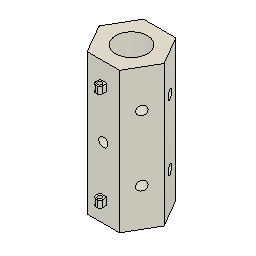
Pen_Holder (Autodesk Fusion 360 design; units mm, degrees)
Autodesk Fusion 360 part; units mm, degrees
sketch "Sketch1" plane through (0, 0, 0) normal (0, 1, 0) x (1, 0, 0)
  line L0 (2.3672, -5.715) -> (5.715, -2.3672)
  line L1 (5.715, -2.3672) -> (5.715, 2.3672)
  line L2 (5.715, 2.3672) -> (2.3672, 5.715)
  line L3 (2.3672, 5.715) -> (-2.3672, 5.715)
  line L4 (-2.3672, 5.715) -> (-5.715, 2.3672)
  line L5 (-5.715, 2.3672) -> (-5.715, -2.3672)
  line L6 (-5.715, -2.3672) -> (-2.3672, -5.715)
  line L7 (-2.3672, -5.715) -> (2.3672, -5.715)
  circle A0 centre (0, 0) radius 5.715
  line L8 (5.8659, -10.16) -> (11.7318, 0)
  line L9 (11.7318, 0) -> (5.8659, 10.16)
  line L10 (5.8659, 10.16) -> (-5.8659, 10.16)
  line L11 (-5.8659, 10.16) -> (-11.7318, 0)
  line L12 (-11.7318, 0) -> (-5.8659, -10.16)
  line L13 (-5.8659, -10.16) -> (5.8659, -10.16)
  dimension "d1" = 5.715
  dimension "d2" = 10.16
  constraint coincident A0.centre origin
  constraint tangent L7 A0
  measures "d1" distance of A0.centre L7
  measures "d2" distance of A0.centre L13
extrude "Extrude1" add sketch "Sketch1" along normal blind 50.8 contours L0 L7 A0 | L0 L1 A0 | L6 L7 A0 | L1 L2 A0 | L5 L6 A0 | L2 L3 A0 | L4 L5 A0 | L3 L4 A0 | L8 L9 L10 L11 L12 L13
sketch "Sketch2" plane through (-8.7988, 0, 5.08) normal (-0.866025, 0, 0.5) x (0.5, 0, 0.866025)
  line L0 (-5.8659, 0) -> (5.8659, 0)
  line L1 (5.8659, 0) -> (5.8659, 50.8)
  line L2 (5.8659, 50.8) -> (-5.8659, 50.8)
  line L3 (-5.8659, 50.8) -> (-5.8659, 0)
  line L4 (0, 0) -> (0, 50.8) construction
  circle A0 centre (0, 13.6652) radius 1.651
  circle A1 centre (0, 37.1348) radius 1.651
  dimension "d5" = 3.302
  dimension "d6" = 3.302
  dimension "d7" = 13.6652
  dimension "d8" = 13.6652
  constraint coincident L4.start origin
  constraint midpoint L2 L4.end
  constraint coincident L4 A0.centre
  constraint coincident L4 A1.centre
  measures "d5" diameter of A0
  measures "d6" diameter of A1
  measures "d7" distance of L2 A1.centre
  measures "d8" distance of L0 A0.centre
extrude "Extrude2" cut sketch "Sketch2" against normal blind 8.0264 contours A0 | A1
sketch "Sketch3" plane through (0, 0, 10.16) normal (0, 0, 1) x (1, 0, 0)
  line L0 (-5.8659, 0) -> (5.8659, 0)
  line L1 (5.8659, 0) -> (5.8659, 50.8)
  line L2 (5.8659, 50.8) -> (-5.8659, 50.8)
  line L3 (-5.8659, 50.8) -> (-5.8659, 0)
  line L4 (-1.27, 6.35) -> (1.27, 6.35)
  line L5 (1.27, 6.35) -> (1.27, 8.89)
  line L6 (1.27, 8.89) -> (-1.27, 8.89)
  line L7 (-1.27, 8.89) -> (-1.27, 6.35)
  line L8 (0, 50.8) -> (0, 0) construction
  line L9 (0, 8.89) -> (0, 6.35) construction
  line L10 (-5.8659, 25.4) -> (5.8659, 25.4) construction
  line L11 (1.27, 44.45) -> (1.27, 41.91)
  line L12 (1.27, 41.91) -> (-1.27, 41.91)
  line L13 (-1.27, 44.45) -> (1.27, 44.45)
  line L14 (-1.27, 41.91) -> (-1.27, 44.45)
  dimension "d11" = 2.54
  dimension "d12" = 2.54
  dimension "d13" = 6.35
  constraint horizontal L4
  constraint vertical L5
  constraint horizontal L6
  constraint vertical L7
  constraint midpoint L2 L8.start
  constraint coincident L8.end origin
  constraint midpoint L6 L9.start
  constraint midpoint L4 L9.end
  constraint collinear L8 L9
  constraint midpoint L3 L10.start
  constraint midpoint L1 L10.end
  constraint symmetric L4.start L10 L13.start
  constraint symmetric L4.end L10 L11.start
  constraint symmetric L5.end L10 L11.end
  constraint symmetric L6.end L10 L12.end
  measures "d11" distance of L4.start L4.end
  measures "d12" distance of L4.start L6.end
  measures "d13" distance of L0 L4
extrude "Extrude3" add sketch "Sketch3" along normal blind 2.54 contours L4 L5 L6 L7 | L11 L12 L13 L14
sketch "Sketch4" plane through (0, 6.35, 0) normal (0, -1, 0) x (1, 0, 0)
  line L0 (-1.27, 10.16) -> (1.27, 10.16)
  line L1 (1.27, 10.16) -> (1.27, 12.7)
  line L2 (1.27, 12.7) -> (-1.27, 12.7)
  line L3 (-1.27, 12.7) -> (-1.27, 10.16)
  line L4 (0, 12.7) -> (0, 10.16) construction
  line L5 (-1.27, 11.43) -> (1.27, 11.43)
  circle A0 centre (0, 11.43) radius 0.762
  dimension "d16" = 1.524
  constraint midpoint L2 L4.start
  constraint midpoint L0 L4.end
  constraint midpoint L3 L5.start
  constraint midpoint L1 L5.end
  constraint midpoint L5 A0.centre
  measures "d16" diameter of A0
extrude "Extrude5" cut sketch "Sketch4" against normal blind 65.6107 contours L5 A0 | L5 A0
fillet "Fillet1" radius 0.8382 4 edges at (-1.27, 7.62, 12.7) (1.27, 7.62, 12.7) (-1.27, 43.18, 12.7) (1.27, 43.18, 12.7)
sketch "Sketch5" plane through (-8.7988, 0, -5.08) normal (-0.866025, 0, -0.5) x (-0.5, 0, 0.866025)
  line L0 (-5.8659, 0) -> (5.8659, 0)
  line L1 (5.8659, 0) -> (5.8659, 50.8)
  line L2 (5.8659, 50.8) -> (-5.8659, 50.8)
  line L3 (-5.8659, 50.8) -> (-5.8659, 0)
  line L4 (0, 50.8) -> (0, 0) construction
  line L5 (5.8659, 25.4) -> (-5.8659, 25.4) construction
  line L6 (1.27, 44.45) -> (-1.27, 44.45)
  line L7 (-1.27, 44.45) -> (-1.27, 41.91)
  line L8 (-1.27, 41.91) -> (1.27, 41.91)
  line L9 (1.27, 41.91) -> (1.27, 44.45)
  line L10 (0, 41.91) -> (0, 44.45) construction
  line L11 (-1.27, 8.89) -> (1.27, 8.89)
  line L12 (1.27, 8.89) -> (1.27, 6.35)
  line L13 (1.27, 6.35) -> (-1.27, 6.35)
  line L14 (-1.27, 6.35) -> (-1.27, 8.89)
  dimension "d22" = 2.54
  dimension "d23" = 2.54
  dimension "d24" = 6.35
  constraint midpoint L2 L4.start
  constraint coincident L4.end origin
  constraint midpoint L1 L5.start
  constraint midpoint L3 L5.end
  constraint horizontal L6
  constraint vertical L7
  constraint horizontal L8
  constraint vertical L9
  constraint midpoint L8 L10.start
  constraint midpoint L6 L10.end
  constraint collinear L4 L10
  constraint symmetric L5 L6.start L12.end
  constraint symmetric L5 L6.end L13.end
  constraint symmetric L5 L7.end L11.start
  constraint symmetric L5 L8.end L11.end
  measures "d22" distance of L6.start L8.end
  measures "d23" distance of L7.end L8.end
  measures "d24" distance of L2 L6
extrude "Extrude6" add sketch "Sketch5" along normal blind 2.54 contours L6 L7 L8 L9 | L11 L12 L13 L14
sketch "Sketch6" plane through (0, 44.45, 0) normal (0, 1, 0) x (-1, 0, 0)
  line L0 (9.4338, -3.9801) -> (8.1638, -6.1799)
  line L1 (8.1638, -6.1799) -> (10.3635, -7.4499)
  line L2 (10.3635, -7.4499) -> (11.6335, -5.2501)
  line L3 (11.6335, -5.2501) -> (9.4338, -3.9801)
  line L4 (10.9985, -6.35) -> (8.7988, -5.08) construction
  circle A0 centre (9.8987, -5.715) radius 0.762
  dimension "d27" = 1.524
  constraint midpoint L2 L4.start
  constraint midpoint L0 L4.end
  constraint midpoint L4 A0.centre
  measures "d27" diameter of A0
extrude "Extrude7" cut sketch "Sketch6" against normal blind 45.0178 contours A0
fillet "Fillet2" radius 0.8382 4 edges at (-11.6335, 43.18, -5.2501) (-10.3635, 43.18, -7.4499) (-11.6335, 7.62, -5.2501) (-10.3635, 7.62, -7.4499)
sketch "Sketch7" plane through (8.7988, 0, 5.08) normal (0.866025, 0, 0.5) x (0.5, 0, -0.866025)
  line L0 (-5.8659, 0) -> (5.8659, 0)
  line L1 (5.8659, 0) -> (5.8659, 50.8)
  line L2 (5.8659, 50.8) -> (-5.8659, 50.8)
  line L3 (-5.8659, 50.8) -> (-5.8659, 0)
  line L4 (-3.175, 6.35) -> (3.175, 6.35) construction
  line L5 (3.175, 6.35) -> (3.175, 44.45) construction
  line L6 (3.175, 44.45) -> (-3.175, 44.45) construction
  line L7 (-3.175, 44.45) -> (-3.175, 6.35) construction
  line L8 (-3.175, 25.4) -> (3.175, 25.4) construction
  line L9 (0, 6.35) -> (0, 44.45) construction
  line L10 (-5.8659, 25.4) -> (5.8659, 25.4) construction
  line L11 (0, 50.8) -> (0, 0) construction
  circle A0 centre (0, 13.6525) radius 1.651
  circle A1 centre (0, 37.1475) radius 1.651
  dimension "d31" = 38.1
  dimension "d32" = 6.35
  dimension "d33" = 3.302
  dimension "d34" = 7.3025
  constraint horizontal L4
  constraint vertical L5
  constraint horizontal L6
  constraint vertical L7
  constraint midpoint L7 L8.start
  constraint midpoint L5 L8.end
  constraint midpoint L4 L9.start
  constraint midpoint L6 L9.end
  constraint midpoint L3 L10.start
  constraint midpoint L1 L10.end
  constraint collinear L8 L10
  constraint midpoint L2 L11.start
  constraint coincident L11.end origin
  constraint collinear L9 L11
  constraint coincident L9 A0.centre
  constraint symmetric L8 A0 A1
  measures "d31" distance of L4.end L5.end
  measures "d32" distance of L5.end L6.end
  measures "d33" diameter of A0
  measures "d34" distance of L4 A0.centre
extrude "Extrude8" cut sketch "Sketch7" against normal blind 6.6294 contours A0 | A1
sketch "Sketch8" plane through (8.7988, 0, -5.08) normal (0.866025, 0, -0.5) x (-0.5, 0, -0.866025)
  line L0 (-5.8659, 0) -> (5.8659, 0)
  line L1 (5.8659, 0) -> (5.8659, 50.8)
  line L2 (5.8659, 50.8) -> (-5.8659, 50.8)
  circle A0 centre (0, 37.1475) radius 1.651
  line L3 (-3.175, 44.45) -> (-3.175, 6.35) construction
  line L4 (-3.175, 25.4) -> (3.175, 25.4) construction
  line L5 (3.175, 44.45) -> (-3.175, 44.45) construction
  line L6 (3.175, 6.35) -> (3.175, 44.45) construction
  line L7 (-5.8659, 25.4) -> (5.8659, 25.4) construction
  line L8 (-3.175, 6.35) -> (3.175, 6.35) construction
  line L9 (0, 51.3715) -> (0, 0.9525) construction
  circle A1 centre (0, 13.6525) radius 1.651
  line L10 (0, 6.35) -> (0, 44.45) construction
  line L11 (-5.8659, 0) -> (-5.8659, 50.8)
  line L12 (-5.8659, 25.4) -> (5.8659, 25.4)
  dimension "d37" = 38.1
  dimension "d38" = 6.35
  dimension "d39" = 3.302
  dimension "d40" = 7.3025
  constraint horizontal L8
  constraint vertical L6
  constraint horizontal L5
  constraint vertical L3
  constraint midpoint L4.start L3
  constraint midpoint L4.end L6
  constraint midpoint L10.start L8
  constraint midpoint L10.end L5
  constraint collinear L4 L7
  constraint collinear L9 L10
  constraint coincident A1.centre L10
  constraint symmetric A0 L4 A1
  constraint coincident L0.start L11.start
  constraint coincident L2.end L11.end
  constraint midpoint L11 L7.start
  constraint midpoint L1 L7.end
  constraint collinear L7 L12
  measures "d37" distance of L6.start L5.start
  measures "d38" distance of L5.start L3.start
  measures "d39" diameter of A1
  measures "d40" distance of A1.centre L8
sketch "Sketch9" plane through (0, 0, -10.16) normal (0, 0, -1) x (-1, 0, 0)
  line L0 (-5.8659, 0) -> (5.8659, 0)
  line L1 (5.8659, 0) -> (5.8659, 50.8)
  line L2 (5.8659, 50.8) -> (-5.8659, 50.8)
  line L3 (-5.8659, 50.8) -> (-5.8659, 0)
  circle A0 centre (-0.0893, 37.1475) radius 1.651
  line L4 (-3.2643, 44.45) -> (-3.2643, 6.35) construction
  line L5 (-3.2643, 25.4) -> (3.0857, 25.4) construction
  line L6 (3.0857, 44.45) -> (-3.2643, 44.45) construction
  line L7 (3.0857, 6.35) -> (3.0857, 44.45) construction
  line L8 (-3.2643, 6.35) -> (3.0857, 6.35) construction
  line L9 (-0.0893, 50.419) -> (-0.0893, 0) construction
  circle A1 centre (-0.0893, 13.6525) radius 1.651
  line L10 (-0.0893, 6.35) -> (-0.0893, 44.45) construction
  line L11 (-5.8659, 0) -> (-5.8659, 50.8)
  line L12 (-5.8659, 25.4) -> (5.8659, 25.4)
  dimension "d41" = 38.1
  dimension "d42" = 6.35
  dimension "d43" = 3.302
  dimension "d44" = 7.3025
  constraint horizontal L8
  constraint vertical L7
  constraint horizontal L6
  constraint vertical L4
  constraint midpoint L5.start L4
  constraint midpoint L5.end L7
  constraint midpoint L10.start L8
  constraint midpoint L10.end L6
  constraint collinear L9 L10
  constraint coincident A1.centre L10
  constraint symmetric A0 L5 A1
  constraint coincident L0.start L3.end
  constraint coincident L2.end L3.start
  constraint midpoint L11 L12.start
  constraint midpoint L1 L12.end
  constraint collinear L5 L12
  measures "d41" distance of L7.start L6.start
  measures "d42" distance of L6.start L4.start
  measures "d43" diameter of A1
  measures "d44" distance of A1.centre L8
extrude "Extrude9" cut sketch "Sketch9" against normal blind 11.1506 contours A0 | A1
extrude "Extrude10" cut sketch "Sketch8" against normal blind 6.4516 contours A0 | A1
sketch "Sketch10" plane through (0, 0, 10.16) normal (0, 0, 1) x (1, 0, 0)
  line L0 (-1.27, 41.91) -> (-1.27, 44.45)
  line L1 (-1.27, 44.45) -> (1.27, 44.45)
  line L2 (1.27, 44.45) -> (1.27, 41.91)
  line L3 (1.27, 41.91) -> (-1.27, 41.91)
  line L4 (-1.27, 8.89) -> (1.27, 8.89)
  line L5 (1.27, 8.89) -> (1.27, 6.35)
  line L6 (1.27, 6.35) -> (-1.27, 6.35)
  line L7 (-1.27, 6.35) -> (-1.27, 8.89)
  line L8 (-5.8659, 0) -> (5.8659, 0)
  line L9 (5.8659, 0) -> (5.8659, 50.8)
  line L10 (5.8659, 50.8) -> (-5.8659, 50.8)
  line L11 (-5.8659, 50.8) -> (-5.8659, 0)
  line L12 (0, 0) -> (0, 50.8) construction
  circle A0 centre (0, 25.4) radius 1.651
  dimension "d51" = 3.302
  constraint coincident L12.start origin
  constraint midpoint L10 L12.end
  constraint midpoint L12 A0.centre
  measures "d51" diameter of A0
extrude "Extrude11" cut sketch "Sketch10" against normal blind 8.382 contours A0
sketch "Sketch11" plane through (-8.7988, 0, -5.08) normal (-0.866025, 0, -0.5) x (-0.5, 0, 0.866025)
  line L0 (1.27, 41.91) -> (-1.27, 41.91)
  line L1 (-1.27, 41.91) -> (-1.27, 44.45)
  line L2 (-1.27, 44.45) -> (1.27, 44.45)
  line L3 (1.27, 44.45) -> (1.27, 41.91)
  line L4 (-1.27, 6.35) -> (-1.27, 8.89)
  line L5 (-1.27, 8.89) -> (1.27, 8.89)
  line L6 (1.27, 8.89) -> (1.27, 6.35)
  line L7 (1.27, 6.35) -> (-1.27, 6.35)
  line L8 (-5.8659, 0) -> (5.8659, 0)
  line L9 (5.8659, 0) -> (5.8659, 50.8)
  line L10 (5.8659, 50.8) -> (-5.8659, 50.8)
  line L11 (-5.8659, 50.8) -> (-5.8659, 0)
  line L12 (0, 50.8) -> (0, 0) construction
  circle A0 centre (0, 25.4) radius 1.651
  dimension "d54" = 3.302
  constraint midpoint L10 L12.start
  constraint coincident L12.end origin
  constraint midpoint L12 A0.centre
  measures "d54" diameter of A0
extrude "Extrude12" cut sketch "Sketch11" against normal blind 5.5626 contours A0
equation "d1 = 0.2 in + 0.025 in"
